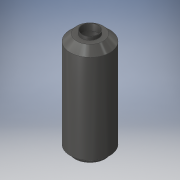
# Autodesk Inventor part: MVX-TL and MVX-TV1X-coarse-reference
Saved by Autodesk Inventor 2016 (Build 200138000, 138)
## iProperties
Created: 2016-07-06
Part Number: MVX-TL and MVX-TV1X-coarse-reference
Material: Generic
Document SubType Name: Modeling
Designer: voigt
Density: 1 g/cm^3
Appearance: Aluminum - Polished(1)
Author: voigt
Autodesk Inventor part; units mm, degrees
ref_plane "YZ Plane" through (0, 0, 0) normal (1, 0, 0) x (0, 1, 0)
ref_plane "XZ Plane" through (0, 0, 0) normal (0, 1, 0) x (-1, 0, 0)
ref_plane "XY Plane" through (0, 0, 0) normal (0, 0, 1) x (1, 0, 0)
sketch "Sketch1" plane through (0, 0, 0) normal (0, 0, 1) x (1, 0, 0)
  circle A0 centre (0, 0) radius 17.75
  circle A1 centre (0, 0) radius 30
  dimension "d0" = 35.5
  dimension "d1" = 60
  constraints: 2 centre point, 2 coincident
  measures "d0" diameter of A0
  measures "d1" diameter of A1
extrude "Extrusion1" add sketch "Sketch1" along normal blind 140
sketch "Sketch2" plane through (0, 0, 0) normal (0, 0, -1) x (-1, 0, 0)
  point P0 (0, 0)
sketch "Sketch3" plane through (0, 0, 0) normal (0, 1, 0) x (-1, 0, 0)
  line L0 (0, -10.8) -> (0, 8.8) construction
  line L1 (-30.85, 0) -> (25.85, 0) construction
  line L2 (-17.75, 140) -> (17.75, 140) construction
  line L3 (17.75, 0) -> (-17.75, 0) construction
  line L4 (-17.75, 0) -> (-17.75, -8)
  line L5 (-17.75, -8) -> (-22.75, -8)
  line L6 (-22.75, -8) -> (-22.75, -6.75)
  line L7 (-17.75, 0) -> (-20.75, 0)
  line L8 (-22.75, -6.75) -> (-20.75, -4.75)
  line L9 (-22.75, -6.75) -> (-19.9216, -6.75) construction
  line L10 (-20.75, -4.75) -> (-20.75, 0)
  point P0 (0, 0)
  dimension "d4" = 8
  dimension "d5" = 5
  dimension "d6" = 1.25
  dimension "d7" = 3
  dimension "d8" = 45
  constraints: 14 end point, 2 perpendicular, 2 vertical, 1 equal length, 1 horizontal, 1 point on line
  measures "d4" distance of L3.end L4.end
  measures "d5" distance of L4.end L5.end
  measures "d6" distance of L5.end L6.end
  measures "d7" distance of L3.end L7.end
  measures "d8" angle of L9 L8
revolve "Revolution1" add sketch "Sketch3" angle 360 about axis through (0, 0, 0) along (0, 0, 1)
sketch "Sketch5" plane through (0, 0, 140) normal (0, 0, 1) x (1, 0, 0)
  circle A0 centre (0, 0) radius 12
  circle A1 centre (0, 0) radius 30 projected
  dimension "d22" = 24
  constraints: 1 centre point, 1 coincident
  measures "d22" diameter of A0
extrude "Extrusion2" add sketch "Sketch5" along normal blind 5
sketch "Sketch6" plane through (0, 0, 145) normal (0, 0, 1) x (1, 0, 0)
  circle A0 centre (0, 0) radius 12 projected
  circle A1 centre (0, 0) radius 12.7
  dimension "d25" = 25.4
  constraints: 1 centre point, 1 coincident
  measures "d25" diameter of A1
extrude "Extrusion3" add sketch "Sketch6" along normal blind 5
chamfer "Chamfer1" distance 10 angle 45 1 edges at (-30, 0, 145)
body "Solid1"
